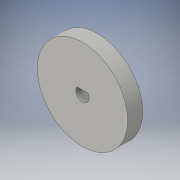
# Autodesk Inventor part: arm4_8
Saved by Autodesk Inventor 2016 (Build 200138000, 138)
## iProperties
Created: 2017-09-20
Part Number: arm4_8
Material: Generic
Document SubType Name: Modeling
Designer: student
Density: 1 g/cm^3
Appearance: Default
Author: student
Autodesk Inventor part; units mm, degrees
ref_plane "YZ Plane" through (0, 0, 0) normal (1, 0, 0) x (0, 1, 0)
ref_plane "XZ Plane" through (0, 0, 0) normal (0, 1, 0) x (-1, 0, 0)
ref_plane "XY Plane" through (0, 0, 0) normal (0, 0, 1) x (1, 0, 0)
sketch "Sketch1" plane through (0, 0, 0) normal (0, 0, 1) x (1, 0, 0)
  circle A0 centre (-808.5404, 25.2471) radius 9.525
  arc A1 (-809.6763, 26.0603) -> (-807.4045, 26.0603) centre (-808.5404, 25.2471) ccw
  line L0 (-808.5404, 23.8501) -> (-808.5404, 26.3901) construction
  line L1 (-807.4045, 26.0603) -> (-809.6763, 26.0603)
  point P0 (0, 0)
  dimension "d0" = 19.05
  dimension "d1" = 2.794
  dimension "d2" = 2.54
  constraints: 4 end point, 3 point on circle, 2 centre point, 1 coincident, 1 horizontal, 1 vertical
  measures "d0" diameter of A0
  measures "d1" diameter of A1
  measures "d2" distance of L0.start L0.end
extrude "Extrusion1" add sketch "Sketch1" along normal blind 3.175
body "Solid1"
